Autodesk Fusion 360 part; units mm, degrees
(part 2 of 5)
  spline S15 degree 5 poles (11.8021, 7.5307) (11.7927, 7.5313) (11.774, 7.5325) (11.746, 7.5342) (11.7087, 7.5364) (11.6621, 7.5388) (11.6156, 7.541) (11.5692, 7.5429) (11.5229, 7.5445) (11.4766, 7.5458) (11.4305, 7.5469) (11.3844, 7.5477) (11.3384, 7.5482) (11.2924, 7.5484) (11.2466, 7.5484) (11.2009, 7.5481) (11.1552, 7.5475) (11.1097, 7.5466) (11.0642, 7.5454) (11.0189, 7.544) (10.9736, 7.5423) (10.9285, 7.5403) (10.8834, 7.538) (10.8385, 7.5354) (10.7937, 7.5325) (10.7489, 7.5293) (10.7044, 7.5259) (10.6599, 7.5221) (10.6155, 7.5181) (10.5713, 7.5137) (10.5271, 7.5091) (10.4832, 7.5042) (10.4393, 7.4989) (10.3956, 7.4934) (10.352, 7.4876) (10.3085, 7.4814) (10.2652, 7.475) (10.222, 7.4682) (10.179, 7.4611) (10.1361, 7.4538) (10.0934, 7.4461) (10.0508, 7.438) (10.0084, 7.4297) (9.9662, 7.421) (9.9241, 7.412) (9.8822, 7.4027) (9.8404, 7.393) (9.7989, 7.383) (9.7575, 7.3727) (9.7163, 7.362) (9.6753, 7.351) (9.6345, 7.3396) (9.594, 7.3278) (9.5536, 7.3156) (9.5135, 7.303) (9.4736, 7.2901) (9.4339, 7.2768) (9.3944, 7.2632) (9.3551, 7.2492) (9.3161, 7.2349) (9.2774, 7.22) (9.239, 7.2046) (9.201, 7.1886) (9.1634, 7.172) (9.1261, 7.1549) (9.0891, 7.1374) (9.0523, 7.1196) (9.0157, 7.1016) (8.9794, 7.0831) (8.9437, 7.064) (8.9087, 7.0436) (8.8816, 7.0261) (8.862, 7.012) (8.8491, 7.0022) (8.8428, 6.9972) knots -1 -1 -1 -1 -1 -1 -0.98571429 -0.97142857 -0.95714286 -0.94285714 -0.92857143 -0.91428571 -0.9 -0.88571429 -0.87142857 -0.85714286 -0.84285714 -0.82857143 -0.81428571 -0.8 -0.78571429 -0.77142857 -0.75714286 -0.74285714 -0.72857143 -0.71428571 -0.7 -0.68571429 -0.67142857 -0.65714286 -0.64285714 -0.62857143 -0.61428571 -0.6 -0.58571429 -0.57142857 -0.55714286 -0.54285714 -0.52857143 -0.51428571 -0.5 -0.48571429 -0.47142857 -0.45714286 -0.44285714 -0.42857143 -0.41428571 -0.4 -0.38571429 -0.37142857 -0.35714286 -0.34285714 -0.32857143 -0.31428571 -0.3 -0.28571429 -0.27142857 -0.25714286 -0.24285714 -0.22857143 -0.21428571 -0.2 -0.18571429 -0.17142857 -0.15714286 -0.14285714 -0.12857143 -0.11428571 -0.1 -0.08571429 -0.07142857 -0.05714286 -0.04285714 -0.02857143 -0.01428571 0 0 0 0 0 0
  line L15 (8.8428, 6.9972) -> (8.2343, 6.5164)
  arc A31 (6.8926, 6.609) -> (8.2343, 6.5164) centre (7.6144, 7.3011) ccw
  arc A32 (6.8926, 6.609) -> (6.609, 6.8926) centre (0, 0) ccw
  arc A33 (6.5164, 8.2343) -> (6.609, 6.8926) centre (7.3011, 7.6144) ccw
  line L16 (6.5164, 8.2343) -> (6.9972, 8.8428)
  spline S16 degree 5 poles (6.9972, 8.8428) (7.0022, 8.8491) (7.012, 8.862) (7.0261, 8.8816) (7.0436, 8.9087) (7.064, 8.9437) (7.0831, 8.9794) (7.1016, 9.0157) (7.1196, 9.0523) (7.1374, 9.0891) (7.1549, 9.1261) (7.172, 9.1634) (7.1886, 9.201) (7.2046, 9.239) (7.22, 9.2774) (7.2349, 9.3161) (7.2492, 9.3551) (7.2632, 9.3944) (7.2768, 9.4339) (7.2901, 9.4736) (7.303, 9.5135) (7.3156, 9.5536) (7.3278, 9.594) (7.3396, 9.6345) (7.351, 9.6753) (7.362, 9.7163) (7.3727, 9.7575) (7.383, 9.7989) (7.393, 9.8404) (7.4027, 9.8822) (7.412, 9.9241) (7.421, 9.9662) (7.4297, 10.0084) (7.438, 10.0508) (7.4461, 10.0934) (7.4538, 10.1361) (7.4611, 10.179) (7.4682, 10.222) (7.475, 10.2652) (7.4814, 10.3085) (7.4876, 10.352) (7.4934, 10.3956) (7.4989, 10.4393) (7.5042, 10.4832) (7.5091, 10.5271) (7.5137, 10.5713) (7.5181, 10.6155) (7.5221, 10.6599) (7.5259, 10.7044) (7.5293, 10.7489) (7.5325, 10.7937) (7.5354, 10.8385) (7.538, 10.8834) (7.5403, 10.9285) (7.5423, 10.9736) (7.544, 11.0189) (7.5454, 11.0642) (7.5466, 11.1097) (7.5475, 11.1552) (7.5481, 11.2009) (7.5484, 11.2466) (7.5484, 11.2924) (7.5482, 11.3384) (7.5477, 11.3844) (7.5469, 11.4305) (7.5458, 11.4766) (7.5445, 11.5229) (7.5429, 11.5692) (7.541, 11.6156) (7.5388, 11.6621) (7.5364, 11.7087) (7.5342, 11.746) (7.5325, 11.774) (7.5313, 11.7927) (7.5307, 11.8021) knots 0 0 0 0 0 0 0.01428571 0.02857143 0.04285714 0.05714286 0.07142857 0.08571429 0.1 0.11428571 0.12857143 0.14285714 0.15714286 0.17142857 0.18571429 0.2 0.21428571 0.22857143 0.24285714 0.25714286 0.27142857 0.28571429 0.3 0.31428571 0.32857143 0.34285714 0.35714286 0.37142857 0.38571429 0.4 0.41428571 0.42857143 0.44285714 0.45714286 0.47142857 0.48571429 0.5 0.51428571 0.52857143 0.54285714 0.55714286 0.57142857 0.58571429 0.6 0.61428571 0.62857143 0.64285714 0.65714286 0.67142857 0.68571429 0.7 0.71428571 0.72857143 0.74285714 0.75714286 0.77142857 0.78571429 0.8 0.81428571 0.82857143 0.84285714 0.85714286 0.87142857 0.88571429 0.9 0.91428571 0.92857143 0.94285714 0.95714286 0.97142857 0.98571429 1 1 1 1 1 1
  arc A34 (7.5307, 11.8021) -> (6.4556, 12.4228) centre (0, 0) ccw
  spline S17 degree 5 poles (6.4556, 12.4228) (6.4472, 12.4186) (6.4304, 12.4104) (6.4052, 12.3979) (6.3718, 12.3811) (6.3303, 12.3599) (6.2889, 12.3385) (6.2478, 12.3169) (6.2069, 12.2952) (6.1661, 12.2732) (6.1256, 12.251) (6.0853, 12.2287) (6.0452, 12.2061) (6.0053, 12.1834) (5.9656, 12.1604) (5.9262, 12.1373) (5.887, 12.1139) (5.848, 12.0904) (5.8092, 12.0667) (5.7706, 12.0427) (5.7323, 12.0186) (5.6942, 11.9943) (5.6563, 11.9698) (5.6187, 11.9451) (5.5813, 11.9202) (5.5442, 11.8951) (5.5073, 11.8698) (5.4707, 11.8443) (5.4343, 11.8186) (5.3981, 11.7927) (5.3622, 11.7666) (5.3266, 11.7404) (5.2912, 11.7139) (5.2561, 11.6873) (5.2213, 11.6604) (5.1867, 11.6334) (5.1524, 11.6061) (5.1184, 11.5787) (5.0847, 11.551) (5.0512, 11.5232) (5.0181, 11.4952) (4.9852, 11.4669) (4.9527, 11.4385) (4.9204, 11.4099) (4.8885, 11.381) (4.8569, 11.352) (4.8256, 11.3227) (4.7946, 11.2933) (4.7639, 11.2637) (4.7336, 11.2338) (4.7036, 11.2038) (4.674, 11.1735) (4.6447, 11.143) (4.6159, 11.1123) (4.5874, 11.0814) (4.5593, 11.0502) (4.5316, 11.0189) (4.5042, 10.9873) (4.4772, 10.9556) (4.4505, 10.9236) (4.4244, 10.8914) (4.3989, 10.8589) (4.374, 10.826) (4.3497, 10.7929) (4.326, 10.7594) (4.3027, 10.7258) (4.2797, 10.692) (4.2571, 10.658) (4.2349, 10.6239) (4.2134, 10.5894) (4.1933, 10.5543) (4.1787, 10.5256) (4.1687, 10.5035) (4.1625, 10.4886) (4.1595, 10.4811) knots -1 -1 -1 -1 -1 -1 -0.98571429 -0.97142857 -0.95714286 -0.94285714 -0.92857143 -0.91428571 -0.9 -0.88571429 -0.87142857 -0.85714286 -0.84285714 -0.82857143 -0.81428571 -0.8 -0.78571429 -0.77142857 -0.75714286 -0.74285714 -0.72857143 -0.71428571 -0.7 -0.68571429 -0.67142857 -0.65714286 -0.64285714 -0.62857143 -0.61428571 -0.6 -0.58571429 -0.57142857 -0.55714286 -0.54285714 -0.52857143 -0.51428571 -0.5 -0.48571429 -0.47142857 -0.45714286 -0.44285714 -0.42857143 -0.41428571 -0.4 -0.38571429 -0.37142857 -0.35714286 -0.34285714 -0.32857143 -0.31428571 -0.3 -0.28571429 -0.27142857 -0.25714286 -0.24285714 -0.22857143 -0.21428571 -0.2 -0.18571429 -0.17142857 -0.15714286 -0.14285714 -0.12857143 -0.11428571 -0.1 -0.08571429 -0.07142857 -0.05714286 -0.04285714 -0.02857143 -0.01428571 0 0 0 0 0 0
  line L17 (4.1595, 10.4811) -> (3.8729, 9.7605)
  arc A35 (2.6646, 9.1699) -> (3.8729, 9.7605) centre (2.9437, 10.1302) ccw
  arc A36 (2.6646, 9.1699) -> (2.2773, 9.2737) centre (0, 0) ccw
  arc A37 (1.5263, 10.3893) -> (2.2773, 9.2737) centre (2.5158, 10.2448) ccw
  line L18 (1.5263, 10.3893) -> (1.6383, 11.1567)
  spline S18 degree 5 poles (1.6383, 11.1567) (1.6395, 11.1647) (1.6416, 11.1807) (1.6439, 11.2048) (1.6456, 11.237) (1.6458, 11.2774) (1.6445, 11.318) (1.6423, 11.3587) (1.6396, 11.3994) (1.6366, 11.4401) (1.6333, 11.4809) (1.6295, 11.5218) (1.625, 11.5626) (1.6199, 11.6035) (1.614, 11.6445) (1.6075, 11.6854) (1.6005, 11.7264) (1.5929, 11.7674) (1.585, 11.8084) (1.5766, 11.8494) (1.5678, 11.8905) (1.5587, 11.9315) (1.5491, 11.9725) (1.539, 12.0135) (1.5285, 12.0545) (1.5175, 12.0956) (1.5062, 12.1366) (1.4944, 12.1776) (1.4823, 12.2186) (1.4698, 12.2595) (1.4569, 12.3005) (1.4437, 12.3414) (1.4301, 12.3824) (1.4161, 12.4233) (1.4018, 12.4641) (1.3871, 12.505) (1.372, 12.5458) (1.3566, 12.5866) (1.3409, 12.6274) (1.3248, 12.6681) (1.3084, 12.7088) (1.2917, 12.7495) (1.2746, 12.7902) (1.2572, 12.8308) (1.2395, 12.8713) (1.2215, 12.9119) (1.2031, 12.9523) (1.1844, 12.9928) (1.1654, 13.0332) (1.1461, 13.0735) (1.1265, 13.1138) (1.1066, 13.1541) (1.0863, 13.1943) (1.0658, 13.2345) (1.045, 13.2746) (1.0239, 13.3146) (1.0024, 13.3546) (0.9807, 13.3946) (0.9587, 13.4344) (0.9364, 13.4743) (0.9138, 13.514) (0.8909, 13.5538) (0.8678, 13.5934) (0.8443, 13.633) (0.8206, 13.6725) (0.7966, 13.712) (0.7723, 13.7514) (0.7477, 13.7907) (0.7229, 13.8299) (0.6978, 13.8691) (0.6724, 13.9082) (0.6518, 13.9395) (0.6363, 13.9629) (0.6259, 13.9784) (0.6207, 13.9862) knots 0 0 0 0 0 0 0.01428571 0.02857143 0.04285714 0.05714286 0.07142857 0.08571429 0.1 0.11428571 0.12857143 0.14285714 0.15714286 0.17142857 0.18571429 0.2 0.21428571 0.22857143 0.24285714 0.25714286 0.27142857 0.28571429 0.3 0.31428571 0.32857143 0.34285714 0.35714286 0.37142857 0.38571429 0.4 0.41428571 0.42857143 0.44285714 0.45714286 0.47142857 0.48571429 0.5 0.51428571 0.52857143 0.54285714 0.55714286 0.57142857 0.58571429 0.6 0.61428571 0.62857143 0.64285714 0.65714286 0.67142857 0.68571429 0.7 0.71428571 0.72857143 0.74285714 0.75714286 0.77142857 0.78571429 0.8 0.81428571 0.82857143 0.84285714 0.85714286 0.87142857 0.88571429 0.9 0.91428571 0.92857143 0.94285714 0.95714286 0.97142857 0.98571429 1 1 1 1 1 1
  arc A38 (0.6207, 13.9862) -> (-0.6207, 13.9862) centre (0, 0) ccw
  spline S19 degree 5 poles (-0.6207, 13.9862) (-0.6259, 13.9784) (-0.6363, 13.9629) (-0.6518, 13.9395) (-0.6724, 13.9082) (-0.6978, 13.8691) (-0.7229, 13.8299) (-0.7477, 13.7907) (-0.7723, 13.7514) (-0.7966, 13.712) (-0.8206, 13.6725) (-0.8443, 13.633) (-0.8678, 13.5934) (-0.8909, 13.5538) (-0.9138, 13.514) (-0.9364, 13.4743) (-0.9587, 13.4344) (-0.9807, 13.3946) (-1.0024, 13.3546) (-1.0239, 13.3146) (-1.045, 13.2746) (-1.0658, 13.2345) (-1.0863, 13.1943) (-1.1066, 13.1541) (-1.1265, 13.1138) (-1.1461, 13.0735) (-1.1654, 13.0332) (-1.1844, 12.9928) (-1.2031, 12.9523) (-1.2215, 12.9119) (-1.2395, 12.8713) (-1.2572, 12.8308) (-1.2746, 12.7902) (-1.2917, 12.7495) (-1.3084, 12.7088) (-1.3248, 12.6681) (-1.3409, 12.6274) (-1.3566, 12.5866) (-1.372, 12.5458) (-1.3871, 12.505) (-1.4018, 12.4641) (-1.4161, 12.4233) (-1.4301, 12.3824) (-1.4437, 12.3414) (-1.4569, 12.3005) (-1.4698, 12.2595) (-1.4823, 12.2186) (-1.4944, 12.1776) (-1.5062, 12.1366) (-1.5175, 12.0956) (-1.5285, 12.0545) (-1.539, 12.0135) (-1.5491, 11.9725) (-1.5587, 11.9315) (-1.5678, 11.8905) (-1.5766, 11.8494) (-1.585, 11.8084) (-1.5929, 11.7674) (-1.6005, 11.7264) (-1.6075, 11.6854) (-1.614, 11.6445) (-1.6199, 11.6035) (-1.625, 11.5626) (-1.6295, 11.5218) (-1.6333, 11.4809) (-1.6366, 11.4401) (-1.6396, 11.3994) (-1.6423, 11.3587) (-1.6445, 11.318) (-1.6458, 11.2774) (-1.6456, 11.237) (-1.6439, 11.2048) (-1.6416, 11.1807) (-1.6395, 11.1647) (-1.6383, 11.1567) knots -1 -1 -1 -1 -1 -1 -0.98571429 -0.97142857 -0.95714286 -0.94285714 -0.92857143 -0.91428571 -0.9 -0.88571429 -0.87142857 -0.85714286 -0.84285714 -0.82857143 -0.81428571 -0.8 -0.78571429 -0.77142857 -0.75714286 -0.74285714 -0.72857143 -0.71428571 -0.7 -0.68571429 -0.67142857 -0.65714286 -0.64285714 -0.62857143 -0.61428571 -0.6 -0.58571429 -0.57142857 -0.55714286 -0.54285714 -0.52857143 -0.51428571 -0.5 -0.48571429 -0.47142857 -0.45714286 -0.44285714 -0.42857143 -0.41428571 -0.4 -0.38571429 -0.37142857 -0.35714286 -0.34285714 -0.32857143 -0.31428571 -0.3 -0.28571429 -0.27142857 -0.25714286 -0.24285714 -0.22857143 -0.21428571 -0.2 -0.18571429 -0.17142857 -0.15714286 -0.14285714 -0.12857143 -0.11428571 -0.1 -0.08571429 -0.07142857 -0.05714286 -0.04285714 -0.02857143 -0.01428571 0 0 0 0 0 0
  line L19 (-1.6383, 11.1567) -> (-1.5263, 10.3893)
  arc A39 (-2.2773, 9.2737) -> (-1.5263, 10.3893) centre (-2.5158, 10.2448) ccw
  arc A40 (-2.2773, 9.2737) -> (-2.6646, 9.1699) centre (0, 0) ccw
  arc A41 (-3.8729, 9.7605) -> (-2.6646, 9.1699) centre (-2.9437, 10.1302) ccw
  line L20 (-3.8729, 9.7605) -> (-4.1595, 10.4811)
  spline S20 degree 5 poles (-4.1595, 10.4811) (-4.1625, 10.4886) (-4.1687, 10.5035) (-4.1787, 10.5256) (-4.1933, 10.5543) (-4.2134, 10.5894) (-4.2349, 10.6239) (-4.2571, 10.658) (-4.2797, 10.692) (-4.3027, 10.7258) (-4.326, 10.7594) (-4.3497, 10.7929) (-4.374, 10.826) (-4.3989, 10.8589) (-4.4244, 10.8914) (-4.4505, 10.9236) (-4.4772, 10.9556) (-4.5042, 10.9873) (-4.5316, 11.0189) (-4.5593, 11.0502) (-4.5874, 11.0814) (-4.6159, 11.1123) (-4.6447, 11.143) (-4.674, 11.1735) (-4.7036, 11.2038) (-4.7336, 11.2338) (-4.7639, 11.2637) (-4.7946, 11.2933) (-4.8256, 11.3227) (-4.8569, 11.352) (-4.8885, 11.381) (-4.9204, 11.4099) (-4.9527, 11.4385) (-4.9852, 11.4669) (-5.0181, 11.4952) (-5.0512, 11.5232) (-5.0847, 11.551) (-5.1184, 11.5787) (-5.1524, 11.6061) (-5.1867, 11.6334) (-5.2213, 11.6604) (-5.2561, 11.6873) (-5.2912, 11.7139) (-5.3266, 11.7404) (-5.3622, 11.7666) (-5.3981, 11.7927) (-5.4343, 11.8186) (-5.4707, 11.8443) (-5.5073, 11.8698) (-5.5442, 11.8951) (-5.5813, 11.9202) (-5.6187, 11.9451) (-5.6563, 11.9698) (-5.6942, 11.9943) (-5.7323, 12.0186) (-5.7706, 12.0427) (-5.8092, 12.0667) (-5.848, 12.0904) (-5.887, 12.1139) (-5.9262, 12.1373) (-5.9656, 12.1604) (-6.0053, 12.1834) (-6.0452, 12.2061) (-6.0853, 12.2287) (-6.1256, 12.251) (-6.1661, 12.2732) (-6.2069, 12.2952) (-6.2478, 12.3169) (-6.2889, 12.3385) (-6.3303, 12.3599) (-6.3718, 12.3811) (-6.4052, 12.3979) (-6.4304, 12.4104) (-6.4472, 12.4186) (-6.4556, 12.4228) knots 0 0 0 0 0 0 0.01428571 0.02857143 0.04285714 0.05714286 0.07142857 0.08571429 0.1 0.11428571 0.12857143 0.14285714 0.15714286 0.17142857 0.18571429 0.2 0.21428571 0.22857143 0.24285714 0.25714286 0.27142857 0.28571429 0.3 0.31428571 0.32857143 0.34285714 0.35714286 0.37142857 0.38571429 0.4 0.41428571 0.42857143 0.44285714 0.45714286 0.47142857 0.48571429 0.5 0.51428571 0.52857143 0.54285714 0.55714286 0.57142857 0.58571429 0.6 0.61428571 0.62857143 0.64285714 0.65714286 0.67142857 0.68571429 0.7 0.71428571 0.72857143 0.74285714 0.75714286 0.77142857 0.78571429 0.8 0.81428571 0.82857143 0.84285714 0.85714286 0.87142857 0.88571429 0.9 0.91428571 0.92857143 0.94285714 0.95714286 0.97142857 0.98571429 1 1 1 1 1 1
  arc A42 (-6.4556, 12.4228) -> (-7.5307, 11.8021) centre (0, 0) ccw
  spline S21 degree 5 poles (-7.5307, 11.8021) (-7.5313, 11.7927) (-7.5325, 11.774) (-7.5342, 11.746) (-7.5364, 11.7087) (-7.5388, 11.6621) (-7.541, 11.6156) (-7.5429, 11.5692) (-7.5445, 11.5229) (-7.5458, 11.4766) (-7.5469, 11.4305) (-7.5477, 11.3844) (-7.5482, 11.3384) (-7.5484, 11.2924) (-7.5484, 11.2466) (-7.5481, 11.2009) (-7.5475, 11.1552) (-7.5466, 11.1097) (-7.5454, 11.0642) (-7.544, 11.0189) (-7.5423, 10.9736) (-7.5403, 10.9285) (-7.538, 10.8834) (-7.5354, 10.8385) (-7.5325, 10.7937) (-7.5293, 10.7489) (-7.5259, 10.7044) (-7.5221, 10.6599) (-7.5181, 10.6155) (-7.5137, 10.5713) (-7.5091, 10.5271) (-7.5042, 10.4832) (-7.4989, 10.4393) (-7.4934, 10.3956) (-7.4876, 10.352) (-7.4814, 10.3085) (-7.475, 10.2652) (-7.4682, 10.222) (-7.4611, 10.179) (-7.4538, 10.1361) (-7.4461, 10.0934) (-7.438, 10.0508) (-7.4297, 10.0084) (-7.421, 9.9662) (-7.412, 9.9241) (-7.4027, 9.8822) (-7.393, 9.8404) (-7.383, 9.7989) (-7.3727, 9.7575) (-7.362, 9.7163) (-7.351, 9.6753) (-7.3396, 9.6345) (-7.3278, 9.594) (-7.3156, 9.5536) (-7.303, 9.5135) (-7.2901, 9.4736) (-7.2768, 9.4339) (-7.2632, 9.3944) (-7.2492, 9.3551) (-7.2349, 9.3161) (-7.22, 9.2774) (-7.2046, 9.239) (-7.1886, 9.201) (-7.172, 9.1634) (-7.1549, 9.1261) (-7.1374, 9.0891) (-7.1196, 9.0523) (-7.1016, 9.0157) (-7.0831, 8.9794) (-7.064, 8.9437) (-7.0436, 8.9087) (-7.0261, 8.8816) (-7.012, 8.862) (-7.0022, 8.8491) (-6.9972, 8.8428) knots -1 -1 -1 -1 -1 -1 -0.98571429 -0.97142857 -0.95714286 -0.94285714 -0.92857143 -0.91428571 -0.9 -0.88571429 -0.87142857 -0.85714286 -0.84285714 -0.82857143 -0.81428571 -0.8 -0.78571429 -0.77142857 -0.75714286 -0.74285714 -0.72857143 -0.71428571 -0.7 -0.68571429 -0.67142857 -0.65714286 -0.64285714 -0.62857143 -0.61428571 -0.6 -0.58571429 -0.57142857 -0.55714286 -0.54285714 -0.52857143 -0.51428571 -0.5 -0.48571429 -0.47142857 -0.45714286 -0.44285714 -0.42857143 -0.41428571 -0.4 -0.38571429 -0.37142857 -0.35714286 -0.34285714 -0.32857143 -0.31428571 -0.3 -0.28571429 -0.27142857 -0.25714286 -0.24285714 -0.22857143 -0.21428571 -0.2 -0.18571429 -0.17142857 -0.15714286 -0.14285714 -0.12857143 -0.11428571 -0.1 -0.08571429 -0.07142857 -0.05714286 -0.04285714 -0.02857143 -0.01428571 0 0 0 0 0 0
  line L21 (-6.9972, 8.8428) -> (-6.5164, 8.2343)
  arc A43 (-6.609, 6.8926) -> (-6.5164, 8.2343) centre (-7.3011, 7.6144) ccw
  arc A44 (-6.609, 6.8926) -> (-6.8926, 6.609) centre (0, 0) ccw
  arc A45 (-8.2343, 6.5164) -> (-6.8926, 6.609) centre (-7.6144, 7.3011) ccw
  line L22 (-8.2343, 6.5164) -> (-8.8428, 6.9972)
  spline S22 degree 5 poles (-8.8428, 6.9972) (-8.8491, 7.0022) (-8.862, 7.012) (-8.8816, 7.0261) (-8.9087, 7.0436) (-8.9437, 7.064) (-8.9794, 7.0831) (-9.0157, 7.1016) (-9.0523, 7.1196) (-9.0891, 7.1374) (-9.1261, 7.1549) (-9.1634, 7.172) (-9.201, 7.1886) (-9.239, 7.2046) (-9.2774, 7.22) (-9.3161, 7.2349) (-9.3551, 7.2492) (-9.3944, 7.2632) (-9.4339, 7.2768) (-9.4736, 7.2901) (-9.5135, 7.303) (-9.5536, 7.3156) (-9.594, 7.3278) (-9.6345, 7.3396) (-9.6753, 7.351) (-9.7163, 7.362) (-9.7575, 7.3727) (-9.7989, 7.383) (-9.8404, 7.393) (-9.8822, 7.4027) (-9.9241, 7.412) (-9.9662, 7.421) (-10.0084, 7.4297) (-10.0508, 7.438) (-10.0934, 7.4461) (-10.1361, 7.4538) (-10.179, 7.4611) (-10.222, 7.4682) (-10.2652, 7.475) (-10.3085, 7.4814) (-10.352, 7.4876) (-10.3956, 7.4934) (-10.4393, 7.4989) (-10.4832, 7.5042) (-10.5271, 7.5091) (-10.5713, 7.5137) (-10.6155, 7.5181) (-10.6599, 7.5221) (-10.7044, 7.5259) (-10.7489, 7.5293) (-10.7937, 7.5325) (-10.8385, 7.5354) (-10.8834, 7.538) (-10.9285, 7.5403) (-10.9736, 7.5423) (-11.0189, 7.544) (-11.0642, 7.5454) (-11.1097, 7.5466) (-11.1552, 7.5475) (-11.2009, 7.5481) (-11.2466, 7.5484) (-11.2924, 7.5484) (-11.3384, 7.5482) (-11.3844, 7.5477) (-11.4305, 7.5469) (-11.4766, 7.5458) (-11.5229, 7.5445) (-11.5692, 7.5429) (-11.6156, 7.541) (-11.6621, 7.5388) (-11.7087, 7.5364) (-11.746, 7.5342) (-11.774, 7.5325) (-11.7927, 7.5313) (-11.8021, 7.5307) knots 0 0 0 0 0 0 0.01428571 0.02857143 0.04285714 0.05714286 0.07142857 0.08571429 0.1 0.11428571 0.12857143 0.14285714 0.15714286 0.17142857 0.18571429 0.2 0.21428571 0.22857143 0.24285714 0.25714286 0.27142857 0.28571429 0.3 0.31428571 0.32857143 0.34285714 0.35714286 0.37142857 0.38571429 0.4 0.41428571 0.42857143 0.44285714 0.45714286 0.47142857 0.48571429 0.5 0.51428571 0.52857143 0.54285714 0.55714286 0.57142857 0.58571429 0.6 0.61428571 0.62857143 0.64285714 0.65714286 0.67142857 0.68571429 0.7 0.71428571 0.72857143 0.74285714 0.75714286 0.77142857 0.78571429 0.8 0.81428571 0.82857143 0.84285714 0.85714286 0.87142857 0.88571429 0.9 0.91428571 0.92857143 0.94285714 0.95714286 0.97142857 0.98571429 1 1 1 1 1 1
  arc A46 (-11.8021, 7.5307) -> (-12.4228, 6.4556) centre (0, 0) ccw
  spline S23 degree 5 poles (-12.4228, 6.4556) (-12.4186, 6.4472) (-12.4104, 6.4304) (-12.3979, 6.4052) (-12.3811, 6.3718) (-12.3599, 6.3303) (-12.3385, 6.2889) (-12.3169, 6.2478) (-12.2952, 6.2069) (-12.2732, 6.1661) (-12.251, 6.1256) (-12.2287, 6.0853) (-12.2061, 6.0452) (-12.1834, 6.0053) (-12.1604, 5.9656) (-12.1373, 5.9262) (-12.1139, 5.887) (-12.0904, 5.848) (-12.0667, 5.8092) (-12.0427, 5.7706) (-12.0186, 5.7323) (-11.9943, 5.6942) (-11.9698, 5.6563) (-11.9451, 5.6187) (-11.9202, 5.5813) (-11.8951, 5.5442) (-11.8698, 5.5073) (-11.8443, 5.4707) (-11.8186, 5.4343) (-11.7927, 5.3981) (-11.7666, 5.3622) (-11.7404, 5.3266) (-11.7139, 5.2912) (-11.6873, 5.2561) (-11.6604, 5.2213) (-11.6334, 5.1867) (-11.6061, 5.1524) (-11.5787, 5.1184) (-11.551, 5.0847) (-11.5232, 5.0512) (-11.4952, 5.0181) (-11.4669, 4.9852) (-11.4385, 4.9527) (-11.4099, 4.9204) (-11.381, 4.8885) (-11.352, 4.8569) (-11.3227, 4.8256) (-11.2933, 4.7946) (-11.2637, 4.7639) (-11.2338, 4.7336) (-11.2038, 4.7036) (-11.1735, 4.674) (-11.143, 4.6447) (-11.1123, 4.6159) (-11.0814, 4.5874) (-11.0502, 4.5593) (-11.0189, 4.5316) (-10.9873, 4.5042) (-10.9556, 4.4772) (-10.9236, 4.4505) (-10.8914, 4.4244) (-10.8589, 4.3989) (-10.826, 4.374) (-10.7929, 4.3497) (-10.7594, 4.326) (-10.7258, 4.3027) (-10.692, 4.2797) (-10.658, 4.2571) (-10.6239, 4.2349) (-10.5894, 4.2134) (-10.5543, 4.1933) (-10.5256, 4.1787) (-10.5035, 4.1687) (-10.4886, 4.1625) (-10.4811, 4.1595) knots -1 -1 -1 -1 -1 -1 -0.98571429 -0.97142857 -0.95714286 -0.94285714 -0.92857143 -0.91428571 -0.9 -0.88571429 -0.87142857 -0.85714286 -0.84285714 -0.82857143 -0.81428571 -0.8 -0.78571429 -0.77142857 -0.75714286 -0.74285714 -0.72857143 -0.71428571 -0.7 -0.68571429 -0.67142857 -0.65714286 -0.64285714 -0.62857143 -0.61428571 -0.6 -0.58571429 -0.57142857 -0.55714286 -0.54285714 -0.52857143 -0.51428571 -0.5 -0.48571429 -0.47142857 -0.45714286 -0.44285714 -0.42857143 -0.41428571 -0.4 -0.38571429 -0.37142857 -0.35714286 -0.34285714 -0.32857143 -0.31428571 -0.3 -0.28571429 -0.27142857 -0.25714286 -0.24285714 -0.22857143 -0.21428571 -0.2 -0.18571429 -0.17142857 -0.15714286 -0.14285714 -0.12857143 -0.11428571 -0.1 -0.08571429 -0.07142857 -0.05714286 -0.04285714 -0.02857143 -0.01428571 0 0 0 0 0 0
  line L23 (-10.4811, 4.1595) -> (-9.7605, 3.8729)
  arc A47 (-9.1699, 2.6646) -> (-9.7605, 3.8729) centre (-10.1302, 2.9437) ccw
  circle A48 centre (0, 0) radius 2.5
  circle A49 centre (0, 0) radius 9.5492
  circle A50 centre (0, 0) radius 15.4387
  line L24 (6.8926, -6.609) -> (10.9038, -10.9299)
  line L25 (-2.6646, 9.1699) -> (-4.5624, 14.7492)
  constraint concentric A0 A49
  constraint coincident A16.end A49
  constraint concentric A49 A50
  constraint coincident A20.end A21.end
  constraint coincident A50 L24.end
  constraint coincident A40.end A41.end
  constraint coincident A50 L25.end
extrude "Extrude3" cut sketch "Sketch1 (2)" against normal blind 8 contours A21 L10 S10 A22 S11 L11 A23 A24 A25 L12 S12 A26 S13 L13 A27 A28 A29 L14 S14 A30 S15 L15 A31 A32 A33 L16 S16 A34 S17 L17 A35 A36 A37 L18 S18 A38 S19 L19 A39 A40 A49 A50 L24 L25 | A37 L18 S18 A38 S19 L19 A39 A49 | A33 L16 S16 A34 S17 L17 A35 A49 | A21 L10 S10 A22 S11 L11 A23 A49 | A29 L14 S14 A30 S15 L15 A31 A49 | A25 L12 S12 A26 S13 L13 A27 A49 in component "Spur Gear (12 teeth)"
sketch "Sketch2 (2)" plane through (-5.3679, 7.6662, 53.0756) normal (-0.099601, 0.142244, 0.984808) x (-0.819152, -0.573576, 0)
  arc A0 (-19.0056, 10.2656) -> (-23.806, 28.181) centre (-23.6055, 18.6339) ccw
  arc A1 (-24.8202, 29.0642) -> (-23.806, 28.181) centre (-23.827, 29.1807) ccw
  line L0 (-24.8202, 29.0642) -> (-24.9106, 29.8344)
  spline S0 degree 5 poles (-24.9106, 29.8344) (-24.9115, 29.8424) (-24.9137, 29.8584) (-24.9176, 29.8823) (-24.9243, 29.9139) (-24.9347, 29.953) (-24.9464, 29.9918) (-24.959, 30.0306) (-24.9721, 30.0692) (-24.9856, 30.1078) (-24.9994, 30.1463) (-25.0136, 30.1848) (-25.0285, 30.2231) (-25.044, 30.2613) (-25.0603, 30.2993) (-25.0772, 30.3372) (-25.0946, 30.3749) (-25.1125, 30.4126) (-25.1308, 30.4501) (-25.1495, 30.4876) (-25.1686, 30.525) (-25.1881, 30.5622) (-25.208, 30.5993) (-25.2283, 30.6364) (-25.2491, 30.6733) (-25.2703, 30.7101) (-25.2919, 30.7467) (-25.3138, 30.7833) (-25.3361, 30.8198) (-25.3588, 30.8561) (-25.3818, 30.8923) (-25.4052, 30.9284) (-25.4289, 30.9645) (-25.453, 31.0003) (-25.4775, 31.0361) (-25.5022, 31.0718) (-25.5273, 31.1073) (-25.5528, 31.1427) (-25.5785, 31.1781) (-25.6046, 31.2133) (-25.631, 31.2483) (-25.6577, 31.2833) (-25.6847, 31.3181) (-25.712, 31.3528) (-25.7396, 31.3874) (-25.7675, 31.4219) (-25.7957, 31.4563) (-25.8242, 31.4905) (-25.853, 31.5246) (-25.8821, 31.5586) (-25.9115, 31.5924) (-25.9412, 31.6262) (-25.9711, 31.6598) (-26.0013, 31.6932) (-26.0318, 31.7266) (-26.0626, 31.7598) (-26.0937, 31.7929) (-26.125, 31.8259) (-26.1566, 31.8587) (-26.1884, 31.8914) (-26.2205, 31.924) (-26.2529, 31.9564) (-26.2856, 31.9887) (-26.3185, 32.0209) (-26.3516, 32.0529) (-26.385, 32.0848) (-26.4187, 32.1166) (-26.4526, 32.1482) (-26.4867, 32.1797) (-26.5211, 32.211) (-26.5558, 32.2422) (-26.5837, 32.2671) (-26.6047, 32.2857) (-26.6188, 32.298) (-26.6259, 32.3042) knots 0 0 0 0 0 0 0.01428571 0.02857143 0.04285714 0.05714286 0.07142857 0.08571429 0.1 0.11428571 0.12857143 0.14285714 0.15714286 0.17142857 0.18571429 0.2 0.21428571 0.22857143 0.24285714 0.25714286 0.27142857 0.28571429 0.3 0.31428571 0.32857143 0.34285714 0.35714286 0.37142857 0.38571429 0.4 0.41428571 0.42857143 0.44285714 0.45714286 0.47142857 0.48571429 0.5 0.51428571 0.52857143 0.54285714 0.55714286 0.57142857 0.58571429 0.6 0.61428571 0.62857143 0.64285714 0.65714286 0.67142857 0.68571429 0.7 0.71428571 0.72857143 0.74285714 0.75714286 0.77142857 0.78571429 0.8 0.81428571 0.82857143 0.84285714 0.85714286 0.87142857 0.88571429 0.9 0.91428571 0.92857143 0.94285714 0.95714286 0.97142857 0.98571429 1 1 1 1 1 1
  arc A2 (-26.6259, 32.3042) -> (-27.825, 31.9829) centre (-23.6055, 18.6339) ccw
  spline S1 degree 5 poles (-27.825, 31.9829) (-27.828, 31.974) (-27.834, 31.9563) (-27.8429, 31.9297) (-27.8547, 31.8942) (-27.8691, 31.8498) (-27.8832, 31.8055) (-27.897, 31.7611) (-27.9106, 31.7168) (-27.9239, 31.6725) (-27.9369, 31.6281) (-27.9495, 31.5838) (-27.9619, 31.5395) (-27.9741, 31.4952) (-27.9859, 31.4509) (-27.9974, 31.4067) (-28.0086, 31.3624) (-28.0196, 31.3182) (-28.0302, 31.274) (-28.0406, 31.2298) (-28.0506, 31.1857) (-28.0604, 31.1415) (-28.0698, 31.0974) (-28.0789, 31.0533) (-28.0877, 31.0093) (-28.0963, 30.9653) (-28.1045, 30.9213) (-28.1124, 30.8774) (-28.1199, 30.8335) (-28.1272, 30.7896) (-28.1341, 30.7458) (-28.1408, 30.702) (-28.1471, 30.6583) (-28.153, 30.6147) (-28.1587, 30.571) (-28.164, 30.5275) (-28.169, 30.484) (-28.1736, 30.4405) (-28.1779, 30.3971) (-28.1819, 30.3538) (-28.1855, 30.3105) (-28.1888, 30.2673) (-28.1917, 30.2242) (-28.1942, 30.1811) (-28.1964, 30.1382) (-28.1982, 30.0953) (-28.1997, 30.0525) (-28.2008, 30.0097) (-28.2015, 29.9671) (-28.2019, 29.9245) (-28.2019, 29.8821) (-28.2014, 29.8397) (-28.2005, 29.7975) (-28.1992, 29.7554) (-28.1974, 29.7134) (-28.1953, 29.6715) (-28.1927, 29.6297) (-28.1898, 29.588) (-28.1865, 29.5465) (-28.1827, 29.5051) (-28.1784, 29.4638) (-28.1734, 29.4228) (-28.1678, 29.3819) (-28.1615, 29.3413) (-28.1546, 29.3009) (-28.1473, 29.2606) (-28.1397, 29.2205) (-28.1317, 29.1804) (-28.1233, 29.1406) (-28.114, 29.1011) (-28.1034, 29.062) (-28.0934, 29.0314) (-28.0849, 29.0087) (-28.0788, 28.9938) (-28.0756, 28.9864) knots -1 -1 -1 -1 -1 -1 -0.98571429 -0.97142857 -0.95714286 -0.94285714 -0.92857143 -0.91428571 -0.9 -0.88571429 -0.87142857 -0.85714286 -0.84285714 -0.82857143 -0.81428571 -0.8 -0.78571429 -0.77142857 -0.75714286 -0.74285714 -0.72857143 -0.71428571 -0.7 -0.68571429 -0.67142857 -0.65714286 -0.64285714 -0.62857143 -0.61428571 -0.6 -0.58571429 -0.57142857 -0.55714286 -0.54285714 -0.52857143 -0.51428571 -0.5 -0.48571429 -0.47142857 -0.45714286 -0.44285714 -0.42857143 -0.41428571 -0.4 -0.38571429 -0.37142857 -0.35714286 -0.34285714 -0.32857143 -0.31428571 -0.3 -0.28571429 -0.27142857 -0.25714286 -0.24285714 -0.22857143 -0.21428571 -0.2 -0.18571429 -0.17142857 -0.15714286 -0.14285714 -0.12857143 -0.11428571 -0.1 -0.08571429 -0.07142857 -0.05714286 -0.04285714 -0.02857143 -0.01428571 0 0 0 0 0 0
  line L1 (-28.0756, 28.9864) -> (-27.7687, 28.2741)
  arc A3 (-28.2054, 27.0021) -> (-27.7687, 28.2741) centre (-28.6871, 27.8785) ccw
  arc A4 (-28.2054, 27.0021) -> (-28.5527, 26.8017) centre (-23.6055, 18.6339) ccw
  arc A5 (-29.8726, 27.0595) -> (-28.5527, 26.8017) centre (-29.0708, 27.657) ccw
  line L2 (-29.8726, 27.0595) -> (-30.336, 27.6813)
  spline S2 degree 5 poles (-30.336, 27.6813) (-30.3408, 27.6878) (-30.3507, 27.7006) (-30.366, 27.7193) (-30.3876, 27.7432) (-30.4161, 27.7719) (-30.4457, 27.7997) (-30.476, 27.8269) (-30.5067, 27.8538) (-30.5376, 27.8805) (-30.5689, 27.907) (-30.6004, 27.9332) (-30.6325, 27.9589) (-30.665, 27.9842) (-30.6981, 28.009) (-30.7317, 28.0334) (-30.7656, 28.0574) (-30.8, 28.081) (-30.8346, 28.1044) (-30.8695, 28.1275) (-30.9047, 28.1503) (-30.9402, 28.1729) (-30.976, 28.1951) (-31.0121, 28.2169) (-31.0486, 28.2385) (-31.0853, 28.2598) (-31.1224, 28.2808) (-31.1597, 28.3014) (-31.1972, 28.3218) (-31.235, 28.342) (-31.2731, 28.3618) (-31.3114, 28.3814) (-31.3499, 28.4008) (-31.3887, 28.4198) (-31.4278, 28.4386) (-31.4671, 28.4571) (-31.5066, 28.4753) (-31.5463, 28.4933) (-31.5863, 28.511) (-31.6264, 28.5284) (-31.6668, 28.5456) (-31.7074, 28.5625) (-31.7482, 28.5792) (-31.7892, 28.5956) (-31.8305, 28.6117) (-31.8719, 28.6276) (-31.9135, 28.6433) (-31.9553, 28.6587) (-31.9973, 28.6738) (-32.0395, 28.6887) (-32.0818, 28.7033) (-32.1244, 28.7177) (-32.1671, 28.7318) (-32.21, 28.7457) (-32.2531, 28.7593) (-32.2964, 28.7727) (-32.3398, 28.7858) (-32.3834, 28.7987) (-32.4272, 28.8114) (-32.4711, 28.8238) (-32.5152, 28.8359) (-32.5595, 28.8478) (-32.6039, 28.8595) (-32.6485, 28.8709) (-32.6932, 28.882) (-32.7381, 28.893) (-32.7831, 28.9036) (-32.8283, 28.9141) (-32.8736, 28.9243) (-32.9191, 28.9342) (-32.9647, 28.9439) (-33.0013, 28.9515) (-33.0288, 28.9571) (-33.0472, 28.9607) (-33.0564, 28.9625) knots 0 0 0 0 0 0 0.01428571 0.02857143 0.04285714 0.05714286 0.07142857 0.08571429 0.1 0.11428571 0.12857143 0.14285714 0.15714286 0.17142857 0.18571429 0.2 0.21428571 0.22857143 0.24285714 0.25714286 0.27142857 0.28571429 0.3 0.31428571 0.32857143 0.34285714 0.35714286 0.37142857 0.38571429 0.4 0.41428571 0.42857143 0.44285714 0.45714286 0.47142857 0.48571429 0.5 0.51428571 0.52857143 0.54285714 0.55714286 0.57142857 0.58571429 0.6 0.61428571 0.62857143 0.64285714 0.65714286 0.67142857 0.68571429 0.7 0.71428571 0.72857143 0.74285714 0.75714286 0.77142857 0.78571429 0.8 0.81428571 0.82857143 0.84285714 0.85714286 0.87142857 0.88571429 0.9 0.91428571 0.92857143 0.94285714 0.95714286 0.97142857 0.98571429 1 1 1 1 1 1
  arc A6 (-33.0564, 28.9625) -> (-33.9342, 28.0847) centre (-23.6055, 18.6339) ccw
  spline S3 degree 5 poles (-33.9342, 28.0847) (-33.9324, 28.0755) (-33.9287, 28.0572) (-33.9231, 28.0297) (-33.9156, 27.993) (-33.9059, 27.9474) (-33.8959, 27.902) (-33.8857, 27.8566) (-33.8753, 27.8115) (-33.8646, 27.7664) (-33.8537, 27.7216) (-33.8425, 27.6768) (-33.8311, 27.6323) (-33.8195, 27.5878) (-33.8076, 27.5436) (-33.7954, 27.4995) (-33.783, 27.4556) (-33.7704, 27.4118) (-33.7575, 27.3682) (-33.7444, 27.3248) (-33.731, 27.2815) (-33.7173, 27.2384) (-33.7035, 27.1955) (-33.6893, 27.1528) (-33.675, 27.1102) (-33.6603, 27.0678) (-33.6454, 27.0256) (-33.6303, 26.9836) (-33.6149, 26.9418) (-33.5993, 26.9002) (-33.5834, 26.8588) (-33.5672, 26.8176) (-33.5508, 26.7766) (-33.5342, 26.7358) (-33.5172, 26.6952) (-33.5001, 26.6548) (-33.4826, 26.6146) (-33.4649, 26.5747) (-33.4469, 26.5349) (-33.4287, 26.4954) (-33.4102, 26.4561) (-33.3914, 26.4171) (-33.3724, 26.3783) (-33.3531, 26.3397) (-33.3335, 26.3014) (-33.3136, 26.2634) (-33.2935, 26.2256) (-33.2731, 26.188) (-33.2524, 26.1507) (-33.2314, 26.1137) (-33.2102, 26.0769) (-33.1886, 26.0405) (-33.1667, 26.0044) (-33.1445, 25.9686) (-33.122, 25.9331) (-33.0992, 25.8979) (-33.0761, 25.863) (-33.0527, 25.8283) (-33.029, 25.794) (-33.0051, 25.76) (-32.9807, 25.7265) (-32.9559, 25.6934) (-32.9306, 25.6608) (-32.9048, 25.6288) (-32.8787, 25.5972) (-32.8522, 25.566) (-32.8255, 25.5351) (-32.7986, 25.5044) (-32.7714, 25.4741) (-32.7436, 25.4445) (-32.7149, 25.416) (-32.6909, 25.3944) (-32.6722, 25.379) (-32.6594, 25.3692) (-32.6529, 25.3644) knots -1 -1 -1 -1 -1 -1 -0.98571429 -0.97142857 -0.95714286 -0.94285714 -0.92857143 -0.91428571 -0.9 -0.88571429 -0.87142857 -0.85714286 -0.84285714 -0.82857143 -0.81428571 -0.8 -0.78571429 -0.77142857 -0.75714286 -0.74285714 -0.72857143 -0.71428571 -0.7 -0.68571429 -0.67142857 -0.65714286 -0.64285714 -0.62857143 -0.61428571 -0.6 -0.58571429 -0.57142857 -0.55714286 -0.54285714 -0.52857143 -0.51428571 -0.5 -0.48571429 -0.47142857 -0.45714286 -0.44285714 -0.42857143 -0.41428571 -0.4 -0.38571429 -0.37142857 -0.35714286 -0.34285714 -0.32857143 -0.31428571 -0.3 -0.28571429 -0.27142857 -0.25714286 -0.24285714 -0.22857143 -0.21428571 -0.2 -0.18571429 -0.17142857 -0.15714286 -0.14285714 -0.12857143 -0.11428571 -0.1 -0.08571429 -0.07142857 -0.05714286 -0.04285714 -0.02857143 -0.01428571 0 0 0 0 0 0
  line L3 (-32.6529, 25.3644) -> (-32.0311, 24.901)
  arc A7 (-31.7733, 23.5811) -> (-32.0311, 24.901) centre (-32.6286, 24.0991) ccw
  arc A8 (-31.7733, 23.5811) -> (-31.9738, 23.2338) centre (-23.6055, 18.6339) ccw
  arc A9 (-33.2458, 22.7971) -> (-31.9738, 23.2338) centre (-32.8501, 23.7155) ccw
  line L4 (-33.2458, 22.7971) -> (-33.958, 23.1039)
  spline S4 degree 5 poles (-33.958, 23.1039) (-33.9654, 23.1071) (-33.9804, 23.1133) (-34.003, 23.1218) (-34.0337, 23.1318) (-34.0727, 23.1424) (-34.1122, 23.1516) (-34.1521, 23.16) (-34.1921, 23.168) (-34.2322, 23.1757) (-34.2725, 23.183) (-34.3129, 23.1899) (-34.3536, 23.1962) (-34.3944, 23.2018) (-34.4355, 23.2067) (-34.4767, 23.211) (-34.5181, 23.2148) (-34.5597, 23.2181) (-34.6014, 23.2211) (-34.6431, 23.2236) (-34.685, 23.2258) (-34.727, 23.2275) (-34.7691, 23.2289) (-34.8114, 23.2298) (-34.8537, 23.2302) (-34.8962, 23.2303) (-34.9387, 23.2299) (-34.9814, 23.2292) (-35.0241, 23.2281) (-35.0669, 23.2266) (-35.1098, 23.2248) (-35.1528, 23.2226) (-35.1958, 23.22) (-35.239, 23.2171) (-35.2822, 23.2139) (-35.3254, 23.2102) (-35.3687, 23.2063) (-35.4121, 23.202) (-35.4556, 23.1973) (-35.4991, 23.1923) (-35.5427, 23.187) (-35.5863, 23.1814) (-35.63, 23.1754) (-35.6737, 23.1691) (-35.7175, 23.1625) (-35.7613, 23.1555) (-35.8051, 23.1483) (-35.849, 23.1407) (-35.893, 23.1328) (-35.9369, 23.1246) (-35.9809, 23.1161) (-36.025, 23.1073) (-36.0691, 23.0981) (-36.1132, 23.0887) (-36.1573, 23.079) (-36.2015, 23.0689) (-36.2456, 23.0586) (-36.2898, 23.0479) (-36.3341, 23.037) (-36.3783, 23.0258) (-36.4226, 23.0142) (-36.4669, 23.0024) (-36.5111, 22.9903) (-36.5555, 22.9779) (-36.5998, 22.9652) (-36.6441, 22.9522) (-36.6884, 22.939) (-36.7328, 22.9254) (-36.7771, 22.9116) (-36.8215, 22.8974) (-36.8658, 22.883) (-36.9013, 22.8713) (-36.9279, 22.8624) (-36.9457, 22.8563) (-36.9545, 22.8533) knots 0 0 0 0 0 0 0.01428571 0.02857143 0.04285714 0.05714286 0.07142857 0.08571429 0.1 0.11428571 0.12857143 0.14285714 0.15714286 0.17142857 0.18571429 0.2 0.21428571 0.22857143 0.24285714 0.25714286 0.27142857 0.28571429 0.3 0.31428571 0.32857143 0.34285714 0.35714286 0.37142857 0.38571429 0.4 0.41428571 0.42857143 0.44285714 0.45714286 0.47142857 0.48571429 0.5 0.51428571 0.52857143 0.54285714 0.55714286 0.57142857 0.58571429 0.6 0.61428571 0.62857143 0.64285714 0.65714286 0.67142857 0.68571429 0.7 0.71428571 0.72857143 0.74285714 0.75714286 0.77142857 0.78571429 0.8 0.81428571 0.82857143 0.84285714 0.85714286 0.87142857 0.88571429 0.9 0.91428571 0.92857143 0.94285714 0.95714286 0.97142857 0.98571429 1 1 1 1 1 1
  arc A10 (-36.9545, 22.8533) -> (-37.2758, 21.6542) centre (-23.6055, 18.6339) ccw
  spline S5 degree 5 poles (-37.2758, 21.6542) (-37.2697, 21.6472) (-37.2573, 21.6331) (-37.2387, 21.6121) (-37.2139, 21.5841) (-37.1827, 21.5495) (-37.1513, 21.5151) (-37.1198, 21.4809) (-37.0882, 21.447) (-37.0564, 21.4134) (-37.0245, 21.38) (-36.9925, 21.3468) (-36.9603, 21.3139) (-36.928, 21.2813) (-36.8956, 21.2489) (-36.863, 21.2168) (-36.8303, 21.1849) (-36.7975, 21.1533) (-36.7645, 21.122) (-36.7314, 21.091) (-36.6982, 21.0602) (-36.6649, 21.0297) (-36.6314, 20.9995) (-36.5978, 20.9695) (-36.5641, 20.9399) (-36.5302, 20.9105) (-36.4962, 20.8814) (-36.4621, 20.8526) (-36.4279, 20.8241) (-36.3935, 20.7959) (-36.3591, 20.7679) (-36.3245, 20.7403) (-36.2898, 20.713) (-36.2549, 20.686) (-36.22, 20.6593) (-36.1849, 20.6329) (-36.1497, 20.6069) (-36.1144, 20.5811) (-36.079, 20.5557) (-36.0434, 20.5306) (-36.0078, 20.5058) (-35.972, 20.4814) (-35.9361, 20.4573) (-35.9001, 20.4336) (-35.864, 20.4102) (-35.8277, 20.3872) (-35.7914, 20.3645) (-35.7549, 20.3422) (-35.7184, 20.3202) (-35.6817, 20.2986) (-35.6449, 20.2774) (-35.608, 20.2567) (-35.571, 20.2363) (-35.5339, 20.2164) (-35.4966, 20.1969) (-35.4592, 20.1779) (-35.4218, 20.1592) (-35.3842, 20.1409) (-35.3466, 20.123) (-35.3088, 20.1055) (-35.2709, 20.0886) (-35.2329, 20.0724) (-35.1947, 20.0568) (-35.1564, 20.042) (-35.118, 20.0277) (-35.0794, 20.0139) (-35.0408, 20.0005) (-35.0022, 19.9874) (-34.9635, 19.9748) (-34.9246, 19.963) (-34.8855, 19.9527) (-34.854, 19.946) (-34.8301, 19.942) (-34.8141, 19.9399) (-34.8061, 19.9389) knots -1 -1 -1 -1 -1 -1 -0.98571429 -0.97142857 -0.95714286 -0.94285714 -0.92857143 -0.91428571 -0.9 -0.88571429 -0.87142857 -0.85714286 -0.84285714 -0.82857143 -0.81428571 -0.8 -0.78571429 -0.77142857 -0.75714286 -0.74285714 -0.72857143 -0.71428571 -0.7 -0.68571429 -0.67142857 -0.65714286 -0.64285714 -0.62857143 -0.61428571 -0.6 -0.58571429 -0.57142857 -0.55714286 -0.54285714 -0.52857143 -0.51428571 -0.5 -0.48571429 -0.47142857 -0.45714286 -0.44285714 -0.42857143 -0.41428571 -0.4 -0.38571429 -0.37142857 -0.35714286 -0.34285714 -0.32857143 -0.31428571 -0.3 -0.28571429 -0.27142857 -0.25714286 -0.24285714 -0.22857143 -0.21428571 -0.2 -0.18571429 -0.17142857 -0.15714286 -0.14285714 -0.12857143 -0.11428571 -0.1 -0.08571429 -0.07142857 -0.05714286 -0.04285714 -0.02857143 -0.01428571 0 0 0 0 0 0
  line L5 (-34.8061, 19.9389) -> (-34.0358, 19.8486)
  arc A11 (-33.1526, 18.8344) -> (-34.0358, 19.8486) centre (-34.1524, 18.8554) ccw
  arc A12 (-33.1526, 18.8344) -> (-33.1526, 18.4334) centre (-23.6055, 18.6339) ccw
  arc A13 (-34.0358, 17.4192) -> (-33.1526, 18.4334) centre (-34.1524, 18.4124) ccw
  line L6 (-34.0358, 17.4192) -> (-34.8061, 17.3288)
  spline S6 degree 5 poles (-34.8061, 17.3288) (-34.8141, 17.3279) (-34.8301, 17.3257) (-34.854, 17.3218) (-34.8855, 17.3151) (-34.9246, 17.3047) (-34.9635, 17.293) (-35.0022, 17.2804) (-35.0408, 17.2673) (-35.0794, 17.2538) (-35.118, 17.24) (-35.1564, 17.2258) (-35.1947, 17.2109) (-35.2329, 17.1954) (-35.2709, 17.1791) (-35.3088, 17.1622) (-35.3466, 17.1448) (-35.3842, 17.1269) (-35.4218, 17.1086) (-35.4592, 17.0899) (-35.4966, 17.0708) (-35.5339, 17.0513) (-35.571, 17.0314) (-35.608, 17.0111) (-35.6449, 16.9903) (-35.6817, 16.9691) (-35.7184, 16.9475) (-35.7549, 16.9256) (-35.7914, 16.9033) (-35.8277, 16.8806) (-35.864, 16.8576) (-35.9001, 16.8342) (-35.9361, 16.8104) (-35.972, 16.7864) (-36.0078, 16.7619) (-36.0434, 16.7372) (-36.079, 16.7121) (-36.1144, 16.6866) (-36.1497, 16.6609) (-36.1849, 16.6348) (-36.22, 16.6084) (-36.2549, 16.5817) (-36.2898, 16.5547) (-36.3245, 16.5274) (-36.3591, 16.4998) (-36.3935, 16.4719) (-36.4279, 16.4437) (-36.4621, 16.4152) (-36.4962, 16.3863) (-36.5302, 16.3573) (-36.5641, 16.3279) (-36.5978, 16.2982) (-36.6314, 16.2683) (-36.6649, 16.238) (-36.6982, 16.2075) (-36.7314, 16.1768) (-36.7645, 16.1457) (-36.7975, 16.1144) (-36.8303, 16.0828) (-36.863, 16.051) (-36.8956, 16.0189) (-36.928, 15.9865) (-36.9603, 15.9538) (-36.9925, 15.9209) (-37.0245, 15.8878) (-37.0564, 15.8544) (-37.0882, 15.8207) (-37.1198, 15.7868) (-37.1513, 15.7527) (-37.1827, 15.7183) (-37.2139, 15.6836) (-37.2387, 15.6557) (-37.2573, 15.6346) (-37.2697, 15.6206) (-37.2758, 15.6135) knots 0 0 0 0 0 0 0.01428571 0.02857143 0.04285714 0.05714286 0.07142857 0.08571429 0.1 0.11428571 0.12857143 0.14285714 0.15714286 0.17142857 0.18571429 0.2 0.21428571 0.22857143 0.24285714 0.25714286 0.27142857 0.28571429 0.3 0.31428571 0.32857143 0.34285714 0.35714286 0.37142857 0.38571429 0.4 0.41428571 0.42857143 0.44285714 0.45714286 0.47142857 0.48571429 0.5 0.51428571 0.52857143 0.54285714 0.55714286 0.57142857 0.58571429 0.6 0.61428571 0.62857143 0.64285714 0.65714286 0.67142857 0.68571429 0.7 0.71428571 0.72857143 0.74285714 0.75714286 0.77142857 0.78571429 0.8 0.81428571 0.82857143 0.84285714 0.85714286 0.87142857 0.88571429 0.9 0.91428571 0.92857143 0.94285714 0.95714286 0.97142857 0.98571429 1 1 1 1 1 1
  arc A14 (-37.2758, 15.6135) -> (-36.9545, 14.4144) centre (-23.6055, 18.6339) ccw
  spline S7 degree 5 poles (-36.9545, 14.4144) (-36.9457, 14.4114) (-36.9279, 14.4054) (-36.9013, 14.3965) (-36.8658, 14.3847) (-36.8215, 14.3703) (-36.7771, 14.3562) (-36.7328, 14.3423) (-36.6884, 14.3288) (-36.6441, 14.3155) (-36.5998, 14.3025) (-36.5555, 14.2898) (-36.5111, 14.2774) (-36.4669, 14.2653) (-36.4226, 14.2535) (-36.3783, 14.242) (-36.3341, 14.2307) (-36.2898, 14.2198) (-36.2456, 14.2092) (-36.2015, 14.1988) (-36.1573, 14.1888) (-36.1132, 14.179) (-36.0691, 14.1696) (-36.025, 14.1605) (-35.9809, 14.1517) (-35.9369, 14.1431) (-35.893, 14.1349) (-35.849, 14.127) (-35.8051, 14.1195) (-35.7613, 14.1122) (-35.7175, 14.1053) (-35.6737, 14.0986) (-35.63, 14.0923) (-35.5863, 14.0864) (-35.5427, 14.0807) (-35.4991, 14.0754) (-35.4556, 14.0704) (-35.4121, 14.0658) (-35.3687, 14.0615) (-35.3254, 14.0575) (-35.2822, 14.0539) (-35.239, 14.0506) (-35.1958, 14.0477) (-35.1528, 14.0452) (-35.1098, 14.043) (-35.0669, 14.0412) (-35.0241, 14.0397) (-34.9814, 14.0386) (-34.9387, 14.0379) (-34.8962, 14.0375) (-34.8537, 14.0375) (-34.8114, 14.038) (-34.7691, 14.0389) (-34.727, 14.0402) (-34.685, 14.042) (-34.6431, 14.0441) (-34.6014, 14.0467) (-34.5597, 14.0496) (-34.5181, 14.0529) (-34.4767, 14.0567) (-34.4355, 14.061) (-34.3944, 14.066) (-34.3536, 14.0716) (-34.3129, 14.0779) (-34.2725, 14.0848) (-34.2322, 14.0921) (-34.1921, 14.0997) (-34.1521, 14.1077) (-34.1122, 14.1161) (-34.0727, 14.1254) (-34.0337, 14.136) (-34.003, 14.146) (-33.9804, 14.1545) (-33.9654, 14.1606) (-33.958, 14.1638) knots -1 -1 -1 -1 -1 -1 -0.98571429 -0.97142857 -0.95714286 -0.94285714 -0.92857143 -0.91428571 -0.9 -0.88571429 -0.87142857 -0.85714286 -0.84285714 -0.82857143 -0.81428571 -0.8 -0.78571429 -0.77142857 -0.75714286 -0.74285714 -0.72857143 -0.71428571 -0.7 -0.68571429 -0.67142857 -0.65714286 -0.64285714 -0.62857143 -0.61428571 -0.6 -0.58571429 -0.57142857 -0.55714286 -0.54285714 -0.52857143 -0.51428571 -0.5 -0.48571429 -0.47142857 -0.45714286 -0.44285714 -0.42857143 -0.41428571 -0.4 -0.38571429 -0.37142857 -0.35714286 -0.34285714 -0.32857143 -0.31428571 -0.3 -0.28571429 -0.27142857 -0.25714286 -0.24285714 -0.22857143 -0.21428571 -0.2 -0.18571429 -0.17142857 -0.15714286 -0.14285714 -0.12857143 -0.11428571 -0.1 -0.08571429 -0.07142857 -0.05714286 -0.04285714 -0.02857143 -0.01428571 0 0 0 0 0 0
  line L7 (-33.958, 14.1638) -> (-33.2458, 14.4707)
  arc A15 (-31.9738, 14.034) -> (-33.2458, 14.4707) centre (-32.8501, 13.5523) ccw
  arc A16 (-31.9738, 14.034) -> (-31.7733, 13.6867) centre (-23.6055, 18.6339) ccw
  arc A17 (-32.0311, 12.3668) -> (-31.7733, 13.6867) centre (-32.6286, 13.1686) ccw
  line L8 (-32.0311, 12.3668) -> (-32.6529, 11.9034)
  spline S8 degree 5 poles (-32.6529, 11.9034) (-32.6594, 11.8986) (-32.6722, 11.8887) (-32.6909, 11.8733) (-32.7149, 11.8518) (-32.7436, 11.8233) (-32.7714, 11.7937) (-32.7986, 11.7634) (-32.8255, 11.7327) (-32.8522, 11.7018) (-32.8787, 11.6705) (-32.9048, 11.639) (-32.9306, 11.6069) (-32.9559, 11.5744) (-32.9807, 11.5413) (-33.0051, 11.5077) (-33.029, 11.4738) (-33.0527, 11.4394) (-33.0761, 11.4048) (-33.0992, 11.3699) (-33.122, 11.3347) (-33.1445, 11.2992) (-33.1667, 11.2634) (-33.1886, 11.2273) (-33.2102, 11.1908) (-33.2314, 11.1541) (-33.2524, 11.117) (-33.2731, 11.0797) (-33.2935, 11.0422) (-33.3136, 11.0044) (-33.3335, 10.9663) (-33.3531, 10.928) (-33.3724, 10.8894) (-33.3914, 10.8506) (-33.4102, 10.8116) (-33.4287, 10.7723) (-33.4469, 10.7328) (-33.4649, 10.6931) (-33.4826, 10.6531) (-33.5001, 10.613) (-33.5172, 10.5726) (-33.5342, 10.532) (-33.5508, 10.4912) (-33.5672, 10.4501) (-33.5834, 10.4089) (-33.5993, 10.3675) (-33.6149, 10.3259) (-33.6303, 10.2841) (-33.6454, 10.2421) (-33.6603, 10.1999) (-33.675, 10.1575) (-33.6893, 10.115) (-33.7035, 10.0723) (-33.7173, 10.0293) (-33.731, 9.9863) (-33.7444, 9.943) (-33.7575, 9.8996) (-33.7704, 9.856) (-33.783, 9.8122) (-33.7954, 9.7683) (-33.8076, 9.7242) (-33.8195, 9.6799) (-33.8311, 9.6355) (-33.8425, 9.5909) (-33.8537, 9.5462) (-33.8646, 9.5013) (-33.8753, 9.4563) (-33.8857, 9.4111) (-33.8959, 9.3658) (-33.9059, 9.3203) (-33.9156, 9.2747) (-33.9231, 9.2381) (-33.9287, 9.2106) (-33.9324, 9.1922) (-33.9342, 9.183) knots 0 0 0 0 0 0 0.01428571 0.02857143 0.04285714 0.05714286 0.07142857 0.08571429 0.1 0.11428571 0.12857143 0.14285714 0.15714286 0.17142857 0.18571429 0.2 0.21428571 0.22857143 0.24285714 0.25714286 0.27142857 0.28571429 0.3 0.31428571 0.32857143 0.34285714 0.35714286 0.37142857 0.38571429 0.4 0.41428571 0.42857143 0.44285714 0.45714286 0.47142857 0.48571429 0.5 0.51428571 0.52857143 0.54285714 0.55714286 0.57142857 0.58571429 0.6 0.61428571 0.62857143 0.64285714 0.65714286 0.67142857 0.68571429 0.7 0.71428571 0.72857143 0.74285714 0.75714286 0.77142857 0.78571429 0.8 0.81428571 0.82857143 0.84285714 0.85714286 0.87142857 0.88571429 0.9 0.91428571 0.92857143 0.94285714 0.95714286 0.97142857 0.98571429 1 1 1 1 1 1
  arc A18 (-33.9342, 9.183) -> (-33.0564, 8.3052) centre (-23.6055, 18.6339) ccw
  spline S9 degree 5 poles (-33.0564, 8.3052) (-33.0472, 8.307) (-33.0288, 8.3107) (-33.0013, 8.3163) (-32.9647, 8.3238) (-32.9191, 8.3335) (-32.8736, 8.3435) (-32.8283, 8.3537) (-32.7831, 8.3641) (-32.7381, 8.3748) (-32.6932, 8.3857) (-32.6485, 8.3969) (-32.6039, 8.4083) (-32.5595, 8.4199) (-32.5152, 8.4318) (-32.4711, 8.444) (-32.4272, 8.4564) (-32.3834, 8.469) (-32.3398, 8.4819) (-32.2964, 8.495) (-32.2531, 8.5084) (-32.21, 8.5221) (-32.1671, 8.5359) (-32.1244, 8.5501) (-32.0818, 8.5644) (-32.0395, 8.5791) (-31.9973, 8.594) (-31.9553, 8.6091) (-31.9135, 8.6245) (-31.8719, 8.6401) (-31.8305, 8.656) (-31.7892, 8.6722) (-31.7482, 8.6886) (-31.7074, 8.7052) (-31.6668, 8.7222) (-31.6264, 8.7393) (-31.5863, 8.7568) (-31.5463, 8.7745) (-31.5066, 8.7925) (-31.4671, 8.8107) (-31.4278, 8.8292) (-31.3887, 8.848) (-31.3499, 8.867) (-31.3114, 8.8863) (-31.2731, 8.9059) (-31.235, 8.9258) (-31.1972, 8.9459) (-31.1597, 8.9663) (-31.1224, 8.987) (-31.0853, 9.008) (-31.0486, 9.0292) (-31.0121, 9.0508) (-30.976, 9.0727) (-30.9402, 9.0949) (-30.9047, 9.1174) (-30.8695, 9.1402) (-30.8346, 9.1633) (-30.8, 9.1867) (-30.7656, 9.2104) (-30.7317, 9.2343) (-30.6981, 9.2587) (-30.665, 9.2835) (-30.6325, 9.3088) (-30.6004, 9.3346) (-30.5689, 9.3607) (-30.5376, 9.3872) (-30.5067, 9.4139) (-30.476, 9.4408) (-30.4457, 9.468) (-30.4161, 9.4958) (-30.3876, 9.5245) (-30.366, 9.5485) (-30.3507, 9.5672) (-30.3408, 9.58) (-30.336, 9.5865) knots -1 -1 -1 -1 -1 -1 -0.98571429 -0.97142857 -0.95714286 -0.94285714 -0.92857143 -0.91428571 -0.9 -0.88571429 -0.87142857 -0.85714286 -0.84285714 -0.82857143 -0.81428571 -0.8 -0.78571429 -0.77142857 -0.75714286 -0.74285714 -0.72857143 -0.71428571 -0.7 -0.68571429 -0.67142857 -0.65714286 -0.64285714 -0.62857143 -0.61428571 -0.6 -0.58571429 -0.57142857 -0.55714286 -0.54285714 -0.52857143 -0.51428571 -0.5 -0.48571429 -0.47142857 -0.45714286 -0.44285714 -0.42857143 -0.41428571 -0.4 -0.38571429 -0.37142857 -0.35714286 -0.34285714 -0.32857143 -0.31428571 -0.3 -0.28571429 -0.27142857 -0.25714286 -0.24285714 -0.22857143 -0.21428571 -0.2 -0.18571429 -0.17142857 -0.15714286 -0.14285714 -0.12857143 -0.11428571 -0.1 -0.08571429 -0.07142857 -0.05714286 -0.04285714 -0.02857143 -0.01428571 0 0 0 0 0 0
  line L9 (-30.336, 9.5865) -> (-29.8726, 10.2083)
  arc A19 (-28.5527, 10.4661) -> (-29.8726, 10.2083) centre (-29.0708, 9.6108) ccw
  arc A20 (-28.5527, 10.4661) -> (-28.2054, 10.2656) centre (-23.6055, 18.6339) ccw
  arc A21 (-27.7687, 8.9936) -> (-28.2054, 10.2656) centre (-28.6871, 9.3893) ccw
  line L10 (-27.7687, 8.9936) -> (-28.0756, 8.2814)
  spline S10 degree 5 poles (-28.0756, 8.2814) (-28.0788, 8.274) (-28.0849, 8.259) (-28.0934, 8.2364) (-28.1034, 8.2057) (-28.114, 8.1667) (-28.1233, 8.1271) (-28.1317, 8.0873) (-28.1397, 8.0473) (-28.1473, 8.0071) (-28.1546, 7.9669) (-28.1615, 7.9265) (-28.1678, 7.8858) (-28.1734, 7.845) (-28.1784, 7.8039) (-28.1827, 7.7627) (-28.1865, 7.7213) (-28.1898, 7.6797) (-28.1927, 7.638) (-28.1953, 7.5963) (-28.1974, 7.5544) (-28.1992, 7.5124) (-28.2005, 7.4703) (-28.2014, 7.428) (-28.2019, 7.3857) (-28.2019, 7.3432) (-28.2015, 7.3007) (-28.2008, 7.258) (-28.1997, 7.2153) (-28.1982, 7.1725) (-28.1964, 7.1296) (-28.1942, 7.0866) (-28.1917, 7.0436) (-28.1888, 7.0004) (-28.1855, 6.9572) (-28.1819, 6.914) (-28.1779, 6.8706) (-28.1736, 6.8273) (-28.169, 6.7838) (-28.164, 6.7403) (-28.1587, 6.6967) (-28.153, 6.6531) (-28.1471, 6.6094) (-28.1408, 6.5657) (-28.1341, 6.5219) (-28.1272, 6.4781) (-28.1199, 6.4343) (-28.1124, 6.3904) (-28.1045, 6.3464) (-28.0963, 6.3025) (-28.0877, 6.2584) (-28.0789, 6.2144) (-28.0698, 6.1703) (-28.0604, 6.1262) (-28.0506, 6.0821) (-28.0406, 6.0379) (-28.0302, 5.9938) (-28.0196, 5.9496) (-28.0086, 5.9053) (-27.9974, 5.8611) (-27.9859, 5.8168) (-27.9741, 5.7725) (-27.9619, 5.7282) (-27.9495, 5.6839) (-27.9369, 5.6396) (-27.9239, 5.5953) (-27.9106, 5.551) (-27.897, 5.5066) (-27.8832, 5.4623) (-27.8691, 5.4179) (-27.8547, 5.3736) (-27.8429, 5.3381) (-27.834, 5.3115) (-27.828, 5.2937) (-27.825, 5.2849) knots 0 0 0 0 0 0 0.01428571 0.02857143 0.04285714 0.05714286 0.07142857 0.08571429 0.1 0.11428571 0.12857143 0.14285714 0.15714286 0.17142857 0.18571429 0.2 0.21428571 0.22857143 0.24285714 0.25714286 0.27142857 0.28571429 0.3 0.31428571 0.32857143 0.34285714 0.35714286 0.37142857 0.38571429 0.4 0.41428571 0.42857143 0.44285714 0.45714286 0.47142857 0.48571429 0.5 0.51428571 0.52857143 0.54285714 0.55714286 0.57142857 0.58571429 0.6 0.61428571 0.62857143 0.64285714 0.65714286 0.67142857 0.68571429 0.7 0.71428571 0.72857143 0.74285714 0.75714286 0.77142857 0.78571429 0.8 0.81428571 0.82857143 0.84285714 0.85714286 0.87142857 0.88571429 0.9 0.91428571 0.92857143 0.94285714 0.95714286 0.97142857 0.98571429 1 1 1 1 1 1
  arc A22 (-27.825, 5.2849) -> (-26.6259, 4.9636) centre (-23.6055, 18.6339) ccw